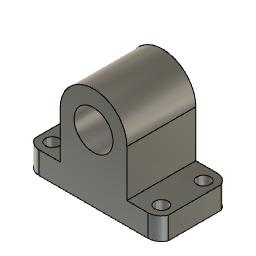
drawing_5 v2 (Autodesk Fusion 360 design; units mm, degrees)
Autodesk Fusion 360 part; units mm, degrees
sketch "Sketch1" plane through (0, 0, 0) normal (0, 0, 1) x (1, 0, 0)
  line L0 (0, 0) -> (-120, 0)
  line L1 (-120, 0) -> (-120, 62)
  line L2 (-120, 62) -> (0, 62)
  line L3 (0, 62) -> (0, 0)
  line L4 (-120, 0) -> (-109, 0)
  line L5 (-120, 62) -> (-109, 62)
  line L6 (0, 62) -> (-11, 62)
  line L7 (0, 0) -> (-11, 0)
  line L8 (-120, 62) -> (-120, 50)
  line L9 (-120, 0) -> (-120, 12)
  line L10 (0, 62) -> (0, 50)
  line L11 (0, 0) -> (0, 12)
  circle A0 centre (-109, 12) radius 6
  circle A1 centre (-109, 12) radius 12
  circle A2 centre (-109, 50) radius 6
  circle A3 centre (-109, 50) radius 12
  circle A4 centre (-11, 50) radius 6
  line L12 (-11, 50) -> (-11, 50.4247)
  circle A5 centre (-11, 50) radius 12
  circle A6 centre (-11, 12) radius 6
  circle A7 centre (-11, 12) radius 12
  dimension "d1" = 120
  dimension "d2" = 62
  dimension "d3" = 11
  dimension "d4" = 11
  dimension "d5" = 11
  dimension "d6" = 11
  dimension "d7" = 12
  dimension "d8" = 12
  dimension "d9" = 12
  dimension "d10" = 12
  dimension "d11" = 12
  dimension "d12" = 24
  dimension "d13" = 12
  dimension "d14" = 24
  dimension "d15" = 12
  dimension "d16" = 24
  dimension "d17" = 12
  dimension "d18" = 24
  constraint horizontal L0
  constraint vertical L1
  constraint horizontal L2
  constraint vertical L3
  constraint coincident L0.start L3.end
  constraint perpendicular L1 L4
  constraint perpendicular L1 L5
  constraint perpendicular L3 L6
  constraint parallel L0 L7
  constraint perpendicular L5 L8
  constraint perpendicular L0 L9
  constraint perpendicular L2 L10
  constraint perpendicular L7 L11
  constraint concentric A0 A1
  constraint concentric A2 A3
  constraint coincident A4.centre L12.start
  constraint vertical L12
  constraint concentric A4 A5
  constraint concentric A6 A7
  measures "d1" distance of L0.start L0.end
  measures "d2" distance of L0.start L2.end
  measures "d3" distance of L0.end L4.end
  measures "d4" distance of L1.end L5.end
  measures "d5" distance of L2.end L6.end
  measures "d6" distance of L0.start L7.end
  measures "d7" distance of L1.end L8.end
  measures "d8" distance of L0.end L9.end
  measures "d9" distance of L2.end L10.end
  measures "d10" distance of L0.start L11.end
  measures "d11" diameter of A0
  measures "d12" diameter of A1
  measures "d13" diameter of A2
  measures "d14" diameter of A3
  measures "d15" diameter of A4
  measures "d16" diameter of A5
  measures "d17" diameter of A6
  measures "d18" diameter of A7
extrude "Extrude1" add sketch "Sketch1" along normal blind 20 contours L0 L1 L2 L3 A1 A3 A5 A7 | L3 L11 A7 | L1 L9 A1 | L3 L10 A5 | L1 L8 A3 picked at (-1.7555, 9.8119) picked at (-118.2445, 14.1881) picked at (-1.7555, 52.1881) picked at (-118.2445, 47.8119)
sketch "Sketch2" plane through (0, 0, 0) normal (0, -1, 0) x (1, 0, 0)
  line L0 (-109, 0) -> (-11, 0)
  line L1 (-11, 0) -> (-11, 20)
  line L2 (-11, 20) -> (-109, 20)
  line L3 (-109, 20) -> (-109, 0)
  line L4 (-109, 20) -> (-11, 20)
  line L5 (-60, 20) -> (-90, 20)
  line L6 (-60, 20) -> (-30, 20)
  line L7 (-90, 20) -> (-90, 62)
  line L8 (-30, 20) -> (-30, 62)
  line L9 (-90, 62) -> (-30, 62)
  dimension "d21" = 30
  dimension "d22" = 30
  dimension "d23" = 42
  dimension "d24" = 42
  constraint coincident L2.end L3.start
  constraint coincident L1.end L2.start
  constraint midpoint L2 L5.start
  constraint perpendicular L1 L5
  constraint parallel L2 L6
  constraint perpendicular L4 L7
  constraint perpendicular L4 L8
  measures "d21" distance of L5.start L5.end
  measures "d22" distance of L5.start L6.end
  measures "d23" distance of L5.end L7.end
  measures "d24" distance of L6.end L8.end
extrude "Extrude2" add sketch "Sketch2" against normal blind 62 contours L2 L4 L5 L6 L7 L8 L9
sketch "Sketch3" plane through (0, 0, 0) normal (0, -1, 0) x (1, 0, 0)
  line L0 (-109, 0) -> (-11, 0)
  line L1 (-11, 0) -> (-11, 20)
  line L2 (-11, 20) -> (-30, 20)
  line L3 (-30, 20) -> (-30, 62)
  line L4 (-30, 62) -> (-90, 62)
  line L5 (-90, 62) -> (-90, 20)
  line L6 (-90, 20) -> (-109, 20)
  line L7 (-109, 20) -> (-109, 0)
  circle A0 centre (-60, 62) radius 30
  line L8 (-90, 62) -> (-30, 62)
  constraint midpoint L4 A0.centre
  constraint coincident L4.end A0
  constraint coincident L4.end L5.start
  constraint coincident L3.end L4.start
extrude "Extrude3" add sketch "Sketch3" against normal blind 62 contours L4 A0 L8 picked at (-62.2252, 71.7493)
sketch "Sketch4" plane through (0, 0, 0) normal (0, -1, 0) x (1, 0, 0)
  line L0 (-109, 0) -> (-11, 0)
  line L1 (-11, 0) -> (-11, 20)
  line L2 (-11, 20) -> (-30, 20)
  line L3 (-30, 20) -> (-30, 62)
  arc A0 (-30, 62) -> (-90, 62) centre (-60, 62) ccw
  line L4 (-90, 62) -> (-90, 20)
  line L5 (-90, 20) -> (-109, 20)
  line L6 (-109, 20) -> (-109, 0)
  circle A1 centre (-60, 59.9304) radius 17.5
  dimension "d29" = 35
  measures "d29" diameter of A1
extrude "Extrude4" cut sketch "Sketch4" against normal blind 50 contours A1
sketch "Sketch5" plane through (0, 50, 0) normal (0, -1, 0) x (1, 0, 0)
  circle A0 centre (-60, 59.9304) radius 17.5
  circle A1 centre (-60, 59.9304) radius 10
  dimension "d32" = 20
  constraint concentric A0 A1
  measures "d32" diameter of A1
extrude "Extrude5" cut sketch "Sketch5" against normal blind 35 contours A1
sketch "Sketch6" plane through (0, 0, 0) normal (0, 0, -1) x (1, 0, 0)
  circle A0 centre (-109, -12) radius 6
  circle A1 centre (-11, -12) radius 6
  circle A2 centre (-11, -50) radius 6
  circle A3 centre (-109, -50) radius 6
  arc A4 (-11, -62) -> (0, -54.7958) centre (-11, -50) ccw
  line L0 (0, -54.7958) -> (0, -7.2042)
  arc A5 (0, -7.2042) -> (-11, 0) centre (-11, -12) ccw
  line L1 (-11, 0) -> (-109, 0)
  arc A6 (-109, 0) -> (-120, -7.2042) centre (-109, -12) ccw
  line L2 (-120, -7.2042) -> (-120, -54.7958)
  arc A7 (-120, -54.7958) -> (-109, -62) centre (-109, -50) ccw
  line L3 (-109, -62) -> (-11, -62)
